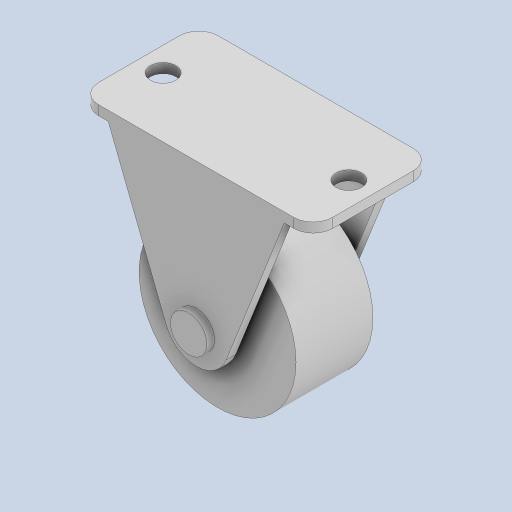
# Autodesk Inventor part: caster
Saved by Autodesk Inventor 2024 (Build 280153000, 153)
## iProperties
Created: 2023-08-07
Part Number: caster
Material: 一般
Document SubType Name: Modeling
Designer: zegi
Density: 1 g/cm^3
Appearance: 既定
Author: zegi
Autodesk Inventor part; units mm, degrees
ref_plane "YZ Plane" through (0, 0, 0) normal (1, 0, 0) x (0, 1, 0)
ref_plane "XZ Plane" through (0, 0, 0) normal (0, 1, 0) x (-1, 0, 0)
ref_plane "XY Plane" through (0, 0, 0) normal (0, 0, 1) x (1, 0, 0)
sketch "スケッチ1" plane through (0, 0, 0) normal (0, 0, 1) x (1, 0, 0)
  circle A0 centre (0, 0) radius 12.25
  circle A1 centre (0, 0) radius 2.85
  circle A2 centre (0, 0) radius 5
  line L0 (4.6517, -1.8335) -> (13.75, 21.25)
  line L1 (0, 0) -> (0, -12.25) construction
  line L2 (0, 21.25) -> (18.25, 21.25)
  line L3 (18.25, 21.25) -> (18.25, 22.75)
  line L4 (18.25, 22.75) -> (0, 22.75)
  line L5 (0, 22.75) -> (0, 21.25)
  line L6 (-4.6517, -1.8335) -> (-13.75, 21.25)
  line L7 (0, 21.25) -> (-18.25, 21.25)
  line L8 (-18.25, 21.25) -> (-18.25, 22.75)
  line L9 (-18.25, 22.75) -> (0, 22.75)
  dimension "d0" = 24.5
  dimension "d2" = 10
  dimension "d1" = 5.7
  dimension "d4" = 1.5
  dimension "d5" = 4.5
  dimension "d6" = 35
  dimension "d7" = 18.25
  constraints: 20 end point, 4 symmetric about line, 3 coincident, 2 parallel, 2 point on line, 2 vertical alignment, 1 centre point, 1 horizontal, 1 perpendicular, 1 vertical, 6 other
  measures "d1" diameter of A1
  measures "d4" distance of L3.end L2.end
  measures "d5" distance of L0.end L2.end
  measures "d6" distance of L1.end L4.end
  measures "d7" distance between parallel lines of L5 L3
extrude "押し出し1" add sketch "スケッチ1" along normal mid plane 12 contours A0 L6 A2 L0 | L0 A2 L6 A0 | A2
extrude "押し出し2" add sketch "スケッチ1" along normal mid plane 21 contours A1
extrude "押し出し3" add sketch "スケッチ1" along normal mid plane 18.65 contours L2 L5 L4 L3 | L7 L8 L9 L5
extrude "押し出し4" add sketch "スケッチ1" against normal blind 1.5 from surface at 9.325 contours L0 A2 L6 A0 | A0 L6 L7 L2 L0 | A2 picked at (-6.2807, 7.4899)
mirror "ミラー1" about plane through (0, 0, 0) normal (0, 0, 1) of "押し出し4"
sketch "スケッチ2" plane through (-18.25, 22.75, -9.325) normal (0, 1, 0) x (1, 0, 0)
  line L0 (36.5, 0) -> (36.5, -18.65) projected
  line L1 (0, 0) -> (36.5, 0) projected
  line L2 (0, -18.65) -> (0, 0) projected
  line L3 (36.5, -18.65) -> (0, -18.65) projected
  line L4 (0, -9.325) -> (36.5, -9.325)
  line L5 (18.25, 0) -> (18.25, -18.65)
  point P0 (18.25, -9.325)
  point P1 (32.75, -9.325)
  point P2 (3.75, -9.325)
  dimension "d25" = 29
  constraints: 4 end point, 4 midpoint, 2 point on line, 1 symmetric about line
  measures "d25" distance of point (3.75, -9.325) point (32.75, -9.325)
hole "穴1" at (14.5, 22.75, 0) at (-14.5, 22.75, 0) direction (0, -1, 0) diameter 4 end through all
fillet "フィレット1" radius 3 4 edges at (-18.25, 22, -9.325) (-18.25, 22, 9.325) (18.25, 22, 9.325) (18.25, 22, -9.325)
